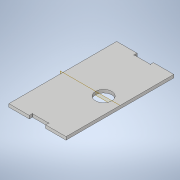
# Autodesk Inventor part: Side_two
Saved by Autodesk Inventor 2020 (Build 240168000, 168)
## iProperties
Created: 2019-12-17
Part Number: Side_two
Material: Generic
Document SubType Name: Modeling
Designer: fabfarm
Density: 1 g/cm^3
Appearance: Default
Author: fabfarm
Autodesk Inventor part; units mm, degrees
ref_plane "YZ Plane" through (0, 0, 0) normal (1, 0, 0) x (0, 1, 0)
ref_plane "XZ Plane" through (0, 0, 0) normal (0, 1, 0) x (-1, 0, 0)
ref_plane "XY Plane" through (0, 0, 0) normal (0, 0, 1) x (1, 0, 0)
sketch "Sketch1" plane through (0, 0, 0) normal (0, 1, 0) x (-1, 0, 0)
  line L0 (0, 0) -> (350, 0)
  line L1 (350, 0) -> (350, 660)
  line L2 (350, 660) -> (0, 660)
  line L3 (0, 660) -> (0, 0)
  dimension "d0" = 350
  dimension "d1" = 660
  constraints: 8 end point, 2 parallel, 1 horizontal, 1 perpendicular
  measures "d0" distance of L0.start L0.end
  measures "d1" distance of L2.end L0.start
extrude "Extrusion1" add sketch "Sketch1" along normal blind 18.55
ref_plane "Work Plane1" through (-350, 0, 330) normal (0, 0, 1) x (1, 0, 0)
sketch "Sketch4" plane through (0, 18.55, 0) normal (0, 1, 0) x (1, 0, 0)
  circle A0 centre (-100, -330) radius 50
  line L0 (70, -330) -> (-420, -330) projected
  line L1 (0, -660) -> (0, 0) projected
  point P0 (0, -641.45)
  point P1 (0, -18.55)
  dimension "d20" = 100
  dimension "d21" = 100
  constraints: 1 centre point, 1 point on line
  measures "d20" diameter of A0
  measures "d21" distance from line of L1 A0.centre
extrude "Extrusion4" cut sketch "Sketch4" against normal blind 20
sketch "Esquisse5" plane through (0, 18.55, 0) normal (0, 1, 0) x (1, 0, 0)
  line L0 (-350, -660) -> (0, -660) projected
  line L1 (-225.1, -660) -> (-124.9, -660)
  line L2 (-124.9, -660) -> (-124.9, -641.45)
  line L3 (-124.9, -641.45) -> (-225.1, -641.45)
  line L4 (-225.1, -641.45) -> (-225.1, -660)
  line L5 (0, 0) -> (-350, 0) projected
  line L6 (-225.1, 0) -> (-124.9, 0)
  line L7 (-124.9, 0) -> (-124.9, -18.55)
  line L8 (-124.9, -18.55) -> (-225.1, -18.55)
  line L9 (-225.1, -18.55) -> (-225.1, 0)
  line L10 (-350, 0) -> (-350, -660) projected
  line L11 (0, -660) -> (0, 0) projected
  point P0 (-124.9, -660)
  dimension "d24" = 100.2
  dimension "d25" = 124.9
  dimension "d26" = 18.55
  dimension "d27" = 18.55
  dimension "d28" = 124.9
  constraints: 16 end point, 4 parallel, 4 point on line, 2 horizontal, 2 perpendicular
  measures "d24" distance of L2.end L3.end
  measures "d25" distance between parallel lines of L10 L4
  measures "d26" distance of L1.end L2.end
  measures "d27" distance of L6.end L7.end
  measures "d28" distance from line of L11 L1.end
extrude "Extrusion5" cut sketch "Esquisse5" against normal blind 100 contours L4 L3 L2 L0 | L5 L7 L8 L9
sketch "Esquisse6" plane through (0, 18.55, 0) normal (0, 1, 0) x (1, 0, 0)
  line L0 (-124.9, -18.55) -> (-225.1, -18.55) projected
  circle A0 centre (-225.1, -18.55) radius 1.585
  circle A1 centre (-124.9, -18.55) radius 1.585
  line L1 (-124.9, -641.45) -> (-225.1, -641.45) projected
  circle A2 centre (-225.1, -641.45) radius 1.585
  circle A3 centre (-124.9, -641.45) radius 1.585
  point P0 (0, 0)
  dimension "d31" = 3.17
  constraints: 4 centre point, 3 equal radius, 2 coincident
  measures "d31" diameter of A3
extrude "Extrusion6" cut sketch "Esquisse6" against normal blind 100
body "Solid1"
